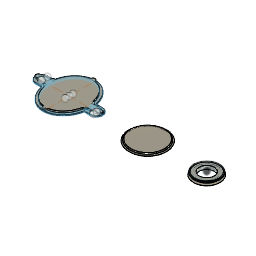
plugs (Autodesk Fusion 360 design; units mm, degrees)
Autodesk Fusion 360 part; units mm, degrees
sketch "Sketch1" plane through (0, 0, 0) normal (0, 0, 1) x (1, 0, 0)
  circle A0 centre (0, 0) radius 20.5
  circle A1 centre (0, 0) radius 24
  dimension "d1" = 41
  dimension "d2" = 48
  constraint coincident A0.centre A1.centre
  measures "d1" diameter of A0
  measures "d2" diameter of A1
extrude "Extrude1" add sketch "Sketch1" along normal blind 3 contours A0 makes body 1
extrude "Extrude2" add sketch "Sketch1" along normal blind 1 bodies 1
sketch "Sketch2" plane through (0, 0, 3) normal (0, 0, 1) x (-1, 0, 0)
  circle A0 centre (0, 0) radius 20.5
  circle A1 centre (0, 0) radius 22.5
  dimension "d7" = 45
  constraint concentric A0 A1
  measures "d7" diameter of A1
extrude "Extrude3" add sketch "Sketch2" against normal blind 1 bodies 1
fillet "Fillet1" radius 1 1 edges at (-22.3759, -8.6788, 0) on bodies 1
chamfer "Chamfer1" distance 1 angle 45 1 edges at (20.9774, 8.1363, 3) on bodies 1
sketch "Sketch3" plane through (0, 0, 0) normal (0, 0, 1) x (1, 0, 0)
  circle A0 centre (75, 0) radius 13
  circle A1 centre (75, 0) radius 17
  dimension "d13" = 26
  dimension "d14" = 34
  constraint concentric A0 A1
  measures "d13" diameter of A0
  measures "d14" diameter of A1
extrude "Extrude4" add sketch "Sketch3" along normal blind 4.5 separate body contours A0 makes body 2
extrude "Extrude5" add sketch "Sketch3" along normal blind 1 bodies 2
sketch "Sketch4" plane through (0, 0, 4.5) normal (0, 0, 1) x (-1, 0, 0)
  circle A0 centre (-75, 0) radius 13
  circle A1 centre (-75, 0) radius 16
  dimension "d19" = 32
  constraint concentric A0 A1
  measures "d19" diameter of A1
extrude "Extrude6" add sketch "Sketch4" against normal blind 1 bodies 2
fillet "Fillet2" radius 1 1 edges at (59.1504, -6.1475, 0) on bodies 2
chamfer "Chamfer2" distance 1 angle 45 1 edges at (89.9172, 5.7858, 4.5) on bodies 2
sketch "Sketch5" plane through (0, 0, 0) normal (0, 0, 1) x (1, 0, 0)
  ellipse E0 centre (-100, 0) end of major axis (-100, 30) minor radius 24.5
  line L0 (-100, -30) -> (-100, 30) construction
  line L1 (-75.5, 0) -> (-124.5, 0) construction
  line L2 (-100, -5) -> (-100, 5)
  circle A0 centre (-65, 0) radius 4
  circle A1 centre (-135, 0) radius 4
  line L3 (-135, 4) -> (-124.2812, 4)
  line L4 (-135, -4) -> (-124.2812, -4)
  line L5 (-65, 4) -> (-75.7188, 4)
  line L6 (-65, -4) -> (-75.7188, -4)
  spline S0 degree 3 poles (-100, -33) (-95.0409, -33) (-90.1038, -31.349) (-85.9117, -28.3548) (-81.1463, -24.951) (-77.3487, -19.8389) (-75.0613, -13.9272) (-72.6061, -7.5814) (-71.8955, -0.328) (-73.0387, 6.5107) (-74.0736, 12.7014) (-76.6194, 18.5381) (-80.3485, 23.1061) (-83.6883, 27.1974) (-87.9791, 30.263) (-92.6862, 31.8159) (-97.2807, 33.3318) (-102.2504, 33.3823) (-106.8681, 31.9582) (-111.935, 30.3955) (-116.5454, 27.082) (-120.0437, 22.6157) (-123.9535, 17.624) (-126.4768, 11.2063) (-127.2437, 4.5025) (-128.0077, -2.1762) (-127.0276, -9.1199) (-124.4445, -15.1387) (-122.1659, -20.4483) (-118.6454, -25.0316) (-114.3089, -28.1955) (-110.2865, -31.1302) (-105.562, -32.8253) (-100.7768, -32.9869) (-100.518, -32.9956) (-100.259, -33) (-100, -33) knots -3.141593 -3.141593 -3.141593 -3.141593 -2.61353 -2.61353 -2.61353 -2.013245 -2.013245 -2.013245 -1.368891 -1.368891 -1.368891 -0.785597 -0.785597 -0.785597 -0.263187 -0.263187 -0.263187 0.246739 0.246739 0.246739 0.806271 0.806271 0.806271 1.43163 1.43163 1.43163 2.054642 2.054642 2.054642 2.60424 2.60424 2.60424 3.114016 3.114016 3.114016 3.141593 3.141593 3.141593 3.141593
  circle A2 centre (-135, 0) radius 7.5
  circle A3 centre (-65, 0) radius 7.5
  line L7 (-65, 7.5) -> (-73.2175, 7.5)
  line L8 (-65, -7.5) -> (-73.2245, -7.5)
  line L9 (-135.0572, 7.5) -> (-126.7805, 7.5)
  line L10 (-135.0572, -7.4998) -> (-126.7629, -7.5631)
  dimension "d25" = 60
  dimension "d26" = 49
  dimension "d30" = 8
  dimension "d31" = 8
  dimension "d32" = 3
  dimension "d33" = 15
  dimension "d34" = 15
  constraint coincident E0 L0.start
  constraint coincident E0 L0.end
  constraint coincident E0 L1.start
  constraint coincident E0 L1.end
  constraint vertical L0
  constraint coincident A1 L3.start
  constraint coincident E0 L3.end
  constraint horizontal L3
  constraint coincident A1 L4.start
  constraint coincident E0 L4.end
  constraint parallel L3 L4
  constraint coincident A0 L5.start
  constraint coincident E0 L5.end
  constraint parallel L4 L5
  constraint coincident E0 L6.end
  constraint parallel L5 L6
  constraint concentric A1 A2
  constraint concentric A0 A3
  constraint coincident A3 L7.start
  constraint coincident S0 L7.end
  constraint horizontal L7
  constraint coincident A3 L8.start
  constraint coincident S0 L8.end
  constraint tangent A3 L8
  constraint coincident S0 L9.end
  constraint parallel L8 L9
  constraint coincident A2 L10.start
  constraint coincident S0 L10.end
  constraint tangent A2 L10
  measures "d25" distance of E0
  measures "d30" diameter of A0
  measures "d31" diameter of A1
  measures "d33" diameter of A2
  measures "d34" diameter of A3
extrude "Extrude8" add sketch "Sketch5" along normal blind 3 separate body contours E0 | E0 L3 L4 S0 | E0 L5 L6 S0 | L3 L4 S0 A2 | L5 L6 S0 A3 | A1 L3 L4 A2 | A0 L5 L6 A3 | A1 | A0 picked at (-129.3916, 2.911) picked at (-71.3049, 0.4501) makes body 3
extrude "Extrude9" add sketch "Sketch5" along normal blind 1 contours E0 L3 L5 S0 | E0 L4 L6 S0 | A1 L3 L4 A2 | L3 S0 A2 L9 | L5 S0 A3 L7 | L4 S0 A2 L10 | L6 S0 A3 L8 | A0 L5 L6 A3 picked at (-135.6075, 6.2878) picked at (-65.3588, 6.3074) bodies 3
sketch "Sketch6" plane through (0, 0, 3) normal (0, 0, 1) x (-1, 0, 0)
  line L0 (65, -4) -> (75.7188, -4)
  ellipse E0 centre (100, 0) end of major axis (100, -30) minor radius 24.5 (75.7188, -4) -> (124.2812, -4) ccw
  line L1 (124.2812, -4) -> (135, -4)
  arc A0 (135, -4) -> (135, 4) centre (135, 0) ccw
  line L2 (135, 4) -> (124.2812, 4)
  ellipse E1 centre (100, 0) end of major axis (100, -30) minor radius 24.5 (124.2812, 4) -> (75.7188, 4) ccw
  line L3 (75.7188, 4) -> (65, 4)
  arc A1 (65, 4) -> (65, -4) centre (65, 0) ccw
  circle A2 centre (100, -30) radius 3
  circle A3 centre (61, 0) radius 3
  circle A4 centre (139, 0) radius 3
  circle A5 centre (100, 30) radius 3
  circle A6 centre (124.2812, -4) radius 3
  circle A7 centre (124.2812, 4) radius 3
  circle A8 centre (75.7188, -4) radius 3
  circle A9 centre (75.7188, 4) radius 3
  point P0 (100, -30)
  dimension "d39" = 6
  dimension "d40" = 6
  dimension "d41" = 6
  dimension "d42" = 6
  dimension "d43" = 6
  constraint coincident P0 A2.centre
  constraint midpoint A1 A3.centre
  constraint midpoint A0 A4.centre
  constraint coincident E1 A5.centre
  constraint coincident L1.start A6.centre
  constraint coincident L2.end A7.centre
  constraint coincident L0.end A8.centre
  constraint coincident L3.start A9.centre
  measures "d39" diameter of A2
  measures "d40" diameter of A6
  measures "d41" diameter of A7
  measures "d42" diameter of A8
  measures "d43" diameter of A9
extrude "Extrude10" add sketch "Sketch6" against normal blind 1 contours L0 E0 A8 | A1 A3 | E0 A2 | E1 L3 A9 | E0 L1 A6 | E1 A5 | A0 A4 | L2 E1 A7 picked at (74.8399, -4.6661) picked at (60.0091, -0.0724) picked at (99.9626, -30.9827) picked at (74.8399, 4.6661) picked at (125.1601, -4.6661) picked at (99.9626, 30.9827) picked at (139.9935, 0) picked at (125.1601, 4.6661) bodies 3
hole "Hole1" at (75, 0, 4.5) direction (0, 0, -1) diameter 19 depth 13 tip angle 118 bodies 2
